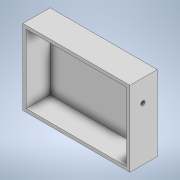
# Autodesk Inventor part: a1
Saved by Autodesk Inventor 2021 (Build 250183000, 183)
## iProperties
Created: 2021-07-11
Part Number: a1
Material: Generic
Document SubType Name: Modeling
Designer: Dell
Density: 1 g/cm^3
Appearance: Default
Author: Dell
Autodesk Inventor part; units mm, degrees
ref_plane "YZ Plane" through (0, 0, 0) normal (1, 0, 0) x (0, 1, 0)
ref_plane "XZ Plane" through (0, 0, 0) normal (0, 1, 0) x (-1, 0, 0)
ref_plane "XY Plane" through (0, 0, 0) normal (0, 0, 1) x (1, 0, 0)
sketch "Sketch1" plane through (0, 0, 0) normal (0, 0, 1) x (1, 0, 0)
  line L0 (0, 13.3457) -> (19.68, 13.3457)
  line L1 (19.68, 13.3457) -> (19.68, -0.5024)
  line L2 (19.68, -0.5024) -> (0, -0.5024)
  line L3 (0, -0.5024) -> (0, 13.3457)
  point P0 (0, 0)
  constraints: 8 end point, 2 parallel, 1 horizontal, 1 perpendicular
extrude "Extrusion1" add sketch "Sketch1" along normal blind 5.0038
shell "Shell1" thickness 0.6 removed faces 1 at (6.56, 4.1137, 5.0038)
sketch "Sketch2" plane through (19.08, 0.0976, 0.6) normal (-1, 0, 0) x (0, 0, 1)
  point P0 (-0.6, -0.0976)
  point P1 (2.0364, 9.2348)
hole "Hole1" at (19.08, 9.3324, 2.6364) direction (1, 0, 0) diameter 0.762 end through all
body "Solid1"
